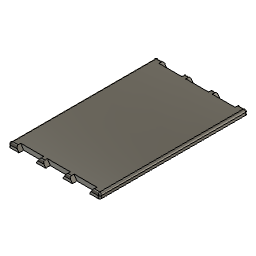
Side Table, Side v4 (Autodesk Fusion 360 design; units mm, degrees)
Autodesk Fusion 360 part; units mm, degrees
sketch "Sketch2" plane through (0, 0, 0) normal (0, 0, 1) x (1, 0, 0)
  line L0 (0, 0) -> (376.7667, 0)
  line L1 (376.7667, 0) -> (376.7667, 609.6)
  line L2 (376.7667, 609.6) -> (0, 609.6)
  line L3 (0, 609.6) -> (0, 0)
  dimension "d4" = 376.7667
  dimension "d5" = 609.6
  constraint horizontal L0
  constraint vertical L1
  constraint horizontal L2
  constraint vertical L3
  constraint coincident L0.start L3.end
  measures "d4" distance of L0.start L0.end
  measures "d5" distance of L0.start L2.end
extrude "Extrude1" add sketch "Sketch2" along normal blind 19.05
sketch "Sketch3" plane through (0, 0, 19.05) normal (0, 0, 1) x (-1, 0, 0)
  line L0 (0, -609.6) -> (0, 0)
  line L1 (0, 0) -> (-376.7667, 0)
  line L2 (-376.7667, 0) -> (-376.7667, -609.6)
  line L3 (-376.7667, -609.6) -> (0, -609.6)
  line L4 (25.4, 0) -> (402.1667, 0)
  line L5 (402.1667, 0) -> (402.1667, -376.7667)
  line L6 (402.1667, -376.7667) -> (25.4, -376.7667)
  line L7 (25.4, -376.7667) -> (25.4, 0)
  dimension "d8" = 376.7667
  dimension "d9" = 376.7667
  constraint horizontal L4
  constraint vertical L5
  constraint horizontal L6
  constraint vertical L7
  measures "d8" distance of L4.start L6.end
  measures "d9" distance of L4.start L4.end
sketch "Sketch4" plane through (0, 0, 19.05) normal (0, 0, 1) x (-1, 0, 0)
  line L0 (0, -609.6) -> (0, 0)
  line L1 (0, 0) -> (-376.7667, 0)
  line L2 (-376.7667, 0) -> (-376.7667, -609.6)
  line L3 (-376.7667, -609.6) -> (0, -609.6)
  line L4 (25.4, 0) -> (71.9667, 0)
  line L5 (25.4, 0) -> (25.4, -25.4)
  line L6 (402.1667, -25.4) -> (402.1667, 0)
  line L7 (402.1667, -25.4) -> (402.1667, 0)
  line L8 (46.587, 0) -> (25.4, 0)
  line L9 (71.9667, 0) -> (56.4444, 0)
  line L10 (56.4444, 0) -> (71.9667, -25.4)
  line L11 (150.9889, 0) -> (135.4667, -25.4)
  line L12 (150.9889, 0) -> (166.5111, 0)
  line L13 (166.5111, 0) -> (182.0333, 0)
  line L14 (166.5111, 0) -> (182.0333, -25.4)
  line L15 (245.5333, -25.4) -> (261.0555, 0)
  line L16 (261.0555, 0) -> (276.5778, 0)
  line L17 (276.5778, 0) -> (292.1, -25.4)
  line L18 (355.6, -25.4) -> (371.1222, 0)
  line L19 (402.1667, 0) -> (386.6444, 0)
  line L20 (386.6444, 0) -> (371.1222, 0)
  line L21 (402.1667, 0) -> (402.1667, -376.7667)
  line L22 (402.1667, -188.3833) -> (25.4, -188.3833)
  line L23 (402.1667, -351.3667) -> (402.1667, -376.7667)
  line L24 (402.1667, -376.7667) -> (402.1667, 0)
  line L25 (166.5111, -376.7667) -> (182.0333, -376.7667)
  line L26 (386.6444, -376.7667) -> (371.1222, -376.7667)
  line L27 (25.4, -376.7667) -> (71.9667, -376.7667)
  line L28 (166.5111, -376.7667) -> (182.0333, -351.3667)
  line L29 (355.6, -351.3667) -> (371.1222, -376.7667)
  line L30 (402.1667, -351.3667) -> (402.1667, -376.7667)
  line L31 (56.4444, -376.7667) -> (71.9667, -351.3667)
  line L32 (245.5333, -351.3667) -> (261.0555, -376.7667)
  line L33 (25.4, -376.7667) -> (25.4, -351.3667)
  line L34 (261.0555, -376.7667) -> (276.5778, -376.7667)
  line L35 (71.9667, -376.7667) -> (56.4444, -376.7667)
  line L36 (46.587, -376.7667) -> (25.4, -376.7667)
  line L37 (276.5778, -376.7667) -> (292.1, -351.3667)
  line L38 (402.1667, -376.7667) -> (386.6444, -376.7667)
  line L39 (150.9889, -376.7667) -> (166.5111, -376.7667)
  line L40 (150.9889, -376.7667) -> (135.4667, -351.3667)
  line L41 (25.4, -25.4) -> (25.4, -19.05)
  line L42 (25.4, -19.05) -> (414.4129, -19.05)
  line L43 (402.1667, -351.3667) -> (402.1667, -357.7167)
  line L44 (402.1667, -357.7167) -> (12.7, -357.7167)
  dimension "d12" = 46.5667
  dimension "d13" = 25.4
  dimension "d14" = 376.7667
  dimension "d15" = 46.5667
  dimension "d16" = 63.5
  dimension "d17" = 46.5667
  dimension "d18" = 15.5222
  dimension "d20" = 15.5222
  dimension "d21" = 15.5222
  dimension "d22" = 63.5
  dimension "d24" = 46.5667
  dimension "d25" = 15.5222
  dimension "d26" = 63.5
  dimension "d456" = 376.7667
  dimension "d473" = 6.35
  dimension "d474" = 6.35
  constraint horizontal L4
  constraint perpendicular L4 L5
  constraint coincident L4 L8.start
  constraint parallel L4 L9
  constraint perpendicular L7 L19
  constraint parallel L19 L20
  constraint perpendicular L19 L21
  constraint midpoint L21 L22.start
  constraint perpendicular L21 L22
  constraint symmetric L4.start L22 L27.start
  constraint symmetric L4.end L22 L27.end
  constraint symmetric L5.end L22 L33.end
  constraint symmetric L6.start L22 L23.start
  constraint symmetric L6.end L22 L21.end
  constraint symmetric L10.end L22 L31.end
  constraint symmetric L8.start L22 L36.start
  constraint symmetric L11.end L22 L40.end
  constraint symmetric L14.end L22 L28.end
  constraint symmetric L9.end L22 L31.start
  constraint symmetric L11.start L22 L39.start
  constraint symmetric L12.end L22 L25.start
  constraint symmetric L13.end L22 L25.end
  constraint symmetric L15.start L22 L32.start
  constraint symmetric L15.end L22 L32.end
  constraint symmetric L17.end L22 L37.end
  constraint symmetric L16.end L22 L34.end
  constraint symmetric L18.start L22 L29.start
  constraint symmetric L18.end L22 L26.end
  constraint symmetric L19.end L22 L26.start
  constraint symmetric L21.end L22 L6.end
  constraint perpendicular L24 L42
  constraint perpendicular L33 L44
  measures "d12" distance of L4.start L4.end
  measures "d13" distance of L4.start L5.end
  measures "d14" distance of L5.end L6.start
  measures "d15" distance of L5.end L10.end
  measures "d16" distance of L10.end L11.end
  measures "d17" distance of L11.end L14.end
  measures "d18" distance of L4.end L9.end
  measures "d20" distance of L11.start L12.end
  measures "d21" distance of L12.end L13.end
  measures "d22" distance of L14.end L15.start
  measures "d24" distance of L15.start L17.end
  measures "d25" distance of L15.end L16.end
  measures "d26" distance of L17.end L18.start
  measures "d456" distance of L6.end L21.end
  measures "d473" distance of L5.end L41.end
  measures "d474" distance of L23.start L43.end
sketch "Sketch5" plane through (0, 609.6, 0) normal (0, 1, 0) x (-1, 0, 0)
  line L0 (-376.7667, 0) -> (0, 0)
  line L1 (0, 0) -> (0, 19.05)
  line L2 (0, 19.05) -> (-376.7667, 19.05)
  line L3 (-376.7667, 19.05) -> (-376.7667, 0)
  line L4 (-376.7667, 0) -> (0, 0)
  line L5 (-123.6562, -70.3757) -> (-108.134, -95.7757)
  line L6 (-328.2673, -70.3757) -> (-343.7895, -70.3757)
  line L7 (-343.7895, -70.3757) -> (-328.2673, -95.7757)
  line L8 (-154.7007, -95.7757) -> (-139.1784, -70.3757)
  line L9 (-233.7229, -70.3757) -> (-218.2007, -95.7757)
  line L10 (-374.834, -95.7757) -> (-328.2673, -95.7757)
  line L11 (-139.1784, -70.3757) -> (-123.6562, -70.3757)
  line L12 (-233.7229, -70.3757) -> (-218.2007, -70.3757)
  line L13 (-249.2451, -70.3757) -> (-264.7673, -95.7757)
  line L14 (-13.5895, -70.3757) -> (-29.1118, -70.3757)
  line L15 (-44.634, -95.7757) -> (-29.1118, -70.3757)
  line L16 (1.9327, -70.3757) -> (-13.5895, -70.3757)
  line L17 (1.9327, -95.7757) -> (1.9327, -70.3757)
  line L18 (-328.2673, -70.3757) -> (-249.2451, -70.3757)
  line L19 (-264.7673, -95.7757) -> (-328.2673, -95.7757)
  line L20 (-218.2007, -95.7757) -> (-154.7007, -95.7757)
  line L21 (-108.134, -95.7757) -> (-44.634, -95.7757)
  line L22 (-29.1118, -70.3757) -> (-123.6562, -70.3757)
  line L23 (-139.1784, -70.3757) -> (-233.7229, -70.3757)
  dimension "d463" = 63.5
  dimension "d464" = 46.5667
  dimension "d465" = 15.5222
  dimension "d466" = 15.5222
  dimension "d467" = 15.5222
  dimension "d468" = 63.5
  dimension "d469" = 46.5667
  dimension "d470" = 15.5222
  dimension "d471" = 63.5
  constraint coincident L0.start L3.end
  constraint coincident L0.end L1.start
  constraint parallel L14 L16
  constraint parallel L10 L19
  constraint parallel L11 L22
  constraint parallel L12 L23
  measures "d463" distance of L13.end L7.end
  measures "d464" distance of L13.end L9.end
  measures "d465" distance of L6.start L6.end
  measures "d466" distance of L9.start L13.start
  measures "d467" distance of L9.start L12.end
  measures "d468" distance of L8.start L9.end
  measures "d469" distance of L8.start L5.end
  measures "d470" distance of L8.end L5.start
  measures "d471" distance of L15.start L5.end
sketch "Sketch6" plane through (0, 0, 0) normal (0, -1, 0) x (1, 0, 0)
  line L0 (0, 0) -> (376.7667, 0)
  line L1 (376.7667, 0) -> (376.7667, 19.05)
  line L2 (376.7667, 19.05) -> (0, 19.05)
  line L3 (0, 19.05) -> (0, 0)
  line L4 (46.5667, 19.05) -> (31.0444, 19.05)
  line L5 (0, -6.35) -> (0, 0)
  line L6 (361.2444, 19.05) -> (345.7222, 19.05)
  line L7 (376.7667, -6.35) -> (376.7667, 19.05)
  line L8 (31.0444, 19.05) -> (46.5667, -6.35)
  line L9 (235.6555, 19.05) -> (251.1778, 19.05)
  line L10 (125.5889, 19.05) -> (141.1111, 19.05)
  line L11 (330.2, -6.35) -> (345.7222, 19.05)
  line L12 (0, 0) -> (389.0129, 0)
  line L13 (125.5889, 19.05) -> (110.0667, -6.35)
  line L14 (376.7667, -6.35) -> (376.7667, 19.05)
  line L15 (376.7667, 19.05) -> (361.2444, 19.05)
  line L16 (0, 19.05) -> (0, -6.35)
  line L17 (0, 19.05) -> (46.5667, 19.05)
  line L18 (220.1333, -6.35) -> (235.6555, 19.05)
  line L19 (21.187, 19.05) -> (0, 19.05)
  line L20 (141.1111, 19.05) -> (156.6333, -6.35)
  line L21 (141.1111, 19.05) -> (156.6333, 19.05)
  line L22 (251.1778, 19.05) -> (266.7, -6.35)
  point P0 (376.7667, 19.05)
  dimension "d492" = 46.5667
  dimension "d493" = 25.4
  dimension "d494" = 376.7667
  dimension "d495" = 46.5667
  dimension "d496" = 63.5
  dimension "d497" = 46.5667
  dimension "d498" = 15.5222
  dimension "d499" = 15.5222
  dimension "d500" = 15.5222
  dimension "d501" = 63.5
  dimension "d502" = 46.5667
  dimension "d503" = 15.5222
  dimension "d504" = 63.5
  dimension "d505" = 6.35
  constraint horizontal L17
  constraint perpendicular L16 L17
  constraint coincident L19.start L17
  constraint parallel L4 L17
  constraint perpendicular L7 L15
  constraint parallel L6 L15
  measures "d492" distance of L4.start L2.end
  measures "d493" distance of L5.start L2.end
  measures "d494" distance of L7.start L5.start
  measures "d495" distance of L8.end L5.start
  measures "d496" distance of L13.end L8.end
  measures "d497" distance of L13.end L20.end
  measures "d498" distance of L4.end L4.start
  measures "d499" distance of L10.start L10.end
  measures "d500" distance of L21.end L10.end
  measures "d501" distance of L18.start L20.end
  measures "d502" distance of L18.start L22.end
  measures "d503" distance of L9.start L9.end
  measures "d504" distance of L11.start L22.end
  measures "d505" distance of L5.start L0.start
fillet "Fillet2" radius 6.35 4 edges at (376.7667, 0, 9.525) (0, 0, 9.525) (376.7667, 609.6, 9.525) (0, 609.6, 9.525)
fillet "Fillet3" radius 8.382 8 edges at (374.9068, 607.7401, 19.05) (188.3833, 609.6, 19.05) (1.8599, 607.7401, 19.05) (0, 304.8, 19.05) (1.8599, 1.8599, 19.05) (188.3833, 0, 19.05) (374.9068, 1.8599, 19.05) (376.7667, 304.8, 19.05)
extrude "Extrude6" cut sketch "Sketch6" against normal blind 19.05 contours L0 L2 L4 L8 L12 L13 L17 | L0 L2 L12 L18 L20 L21 | L0 L2 L11 L12 L22
sketch "Sketch7" plane through (0, 609.6, 0) normal (0, 1, 0) x (-1, 0, 0)
  line L0 (-370.4167, 0) -> (-6.35, 0)
  line L1 (0, 19.05) -> (-376.7667, 19.05)
  line L2 (-376.7667, 19.05) -> (-376.7667, 0)
  line L3 (-355.5797, 19.05) -> (-376.7667, 19.05)
  line L4 (-376.7667, 19.05) -> (-376.7667, -6.35)
  line L5 (-345.7222, 19.05) -> (-330.2, -6.35)
  line L6 (-376.7667, 19.05) -> (-330.2, 19.05)
  line L7 (-376.7667, 0) -> (0, 0)
  line L8 (-330.2, 19.05) -> (-345.7222, 19.05)
  line L9 (-156.6334, -6.35) -> (-141.1111, 19.05)
  line L10 (-251.1778, 19.05) -> (-266.7, -6.35)
  line L11 (-46.5667, -6.35) -> (-31.0445, 19.05)
  line L12 (-141.1111, 19.05) -> (-125.5889, 19.05)
  line L13 (-125.5889, 19.05) -> (-110.0667, -6.35)
  line L14 (-235.6556, 19.05) -> (-220.1333, 19.05)
  line L15 (-251.1778, 19.05) -> (-235.6556, 19.05)
  line L16 (-15.5222, 19.05) -> (-31.0445, 19.05)
  line L17 (0, -6.35) -> (0, 19.05)
  line L18 (0, -6.35) -> (0, 19.05)
  line L19 (-235.6556, 19.05) -> (-220.1334, -6.35)
  line L20 (0, 0) -> (0, 19.05)
  line L21 (0, 19.05) -> (-15.5222, 19.05)
  line L22 (0, 19.05) -> (0, 9.525)
  line L23 (-15.5222, 0) -> (-31.0445, 0)
  line L24 (-330.2, 0) -> (-345.7222, 0)
  line L25 (-235.6556, 0) -> (-220.1333, 0)
  line L26 (-376.7667, 0) -> (-330.2, 0)
  line L27 (-376.7667, 0) -> (-376.7667, 19.05)
  line L28 (-355.5797, 0) -> (-376.7667, 0)
  line L29 (-141.1111, 0) -> (-125.5889, 0)
  line L30 (0, 0) -> (-15.5222, 0)
  line L31 (-251.1778, 0) -> (-235.6556, 0)
  line L32 (0, 0) -> (0, 9.525)
  line L33 (-376.7667, 19.05) -> (0, 19.05)
  line L34 (0, 19.05) -> (0, 0)
  line L35 (-376.7667, 19.05) -> (0, 19.05)
  line L36 (-376.7667, 0) -> (-376.7667, 25.4)
  line L37 (0, 0) -> (-376.7667, 0)
  line L38 (-376.7667, 0) -> (-376.7667, 19.05)
  line L39 (0, 19.05) -> (0, 0)
  line L40 (0, 0) -> (-376.7667, 0)
  line L41 (-6.35, 10.668) -> (-370.4167, 10.668)
  line L42 (-370.4167, 10.668) -> (-370.4167, 0)
  line L43 (-6.35, 0) -> (-6.35, 10.668)
  point P0 (0, 19.05)
  point P1 (-376.7667, 0)
  point P2 (0, 0)
  point P3 (-376.7667, 19.05)
  point P4 (0, 19.05)
  dimension "d522" = 46.5667
  dimension "d523" = 25.4
  dimension "d524" = 376.7667
  dimension "d525" = 46.5667
  dimension "d526" = 63.5
  dimension "d527" = 46.5667
  dimension "d528" = 15.5222
  dimension "d529" = 15.5222
  dimension "d530" = 15.5222
  dimension "d531" = 63.5
  dimension "d532" = 46.5667
  dimension "d533" = 15.5222
  dimension "d534" = 63.5
  constraint horizontal L6
  constraint perpendicular L4 L6
  constraint coincident L3.start L6
  constraint parallel L6 L8
  constraint perpendicular L18 L21
  constraint parallel L16 L21
  constraint coincident P4 P0
  measures "d522" distance of P3 L6.end
  measures "d523" distance of P3 L4.end
  measures "d524" distance of L17.start L4.end
  measures "d525" distance of L5.end L4.end
  measures "d526" distance of L10.end L5.end
  measures "d527" distance of L10.end L19.end
  measures "d528" distance of L5.start L6.end
  measures "d529" distance of L14.start L10.start
  measures "d530" distance of L14.end L14.start
  measures "d531" distance of L9.start L19.end
  measures "d532" distance of L9.start L13.end
  measures "d533" distance of L9.end L12.end
  measures "d534" distance of L11.start L13.end
extrude "Extrude7" cut sketch "Sketch7" against normal blind 19.05 contours L0 L5 L7 L10 L24 L26 L37 L40 L41 | L1 L5 L6 L8 L10 L33 L35 L41 | L0 L7 L9 L19 L25 L37 L40 L41 | L1 L9 L14 L19 L33 L35 L41 | L0 L7 L11 L13 L37 L40 L41 | L1 L11 L13 L33 L35 L41
named bodies: "Side Panel"
